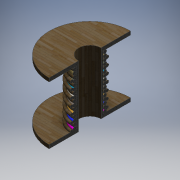
# Autodesk Inventor part: 부품5
Saved by Autodesk Inventor 2016 (Build 200138000, 138)
## iProperties
Created: 2024-06-14
Part Number: 부품5
Material: 강철, 합금
Document SubType Name: Modeling
Designer: pc
Density: 7.73 g/cm^3
Appearance: 내츄럴 단풍나무 - 광택 짙은 착색
Author: pc
Autodesk Inventor part; units mm, degrees
ref_plane "YZ Plane" through (0, 0, 0) normal (1, 0, 0) x (0, 1, 0)
ref_plane "XZ Plane" through (0, 0, 0) normal (0, 1, 0) x (-1, 0, 0)
ref_plane "XY Plane" through (0, 0, 0) normal (0, 0, 1) x (1, 0, 0)
sketch "스케치1" plane through (0, 0, 0) normal (0, 0, 1) x (1, 0, 0)
  circle A0 centre (0, 0) radius 900
  dimension "d0" = 1800
  constraints: 1 centre point, 1 coincident
  measures "d0" diameter of A0
extrude "돌출1" add sketch "스케치1" along normal blind 80
sketch "스케치2" plane through (0, 0, 80) normal (0, 0, 1) x (1, 0, 0)
  circle A0 centre (0, 0) radius 300
  dimension "d3" = 600
  constraints: 1 centre point, 1 coincident
  measures "d3" diameter of A0
extrude "돌출2" add sketch "스케치2" along normal blind 1200
sketch "스케치3" plane through (0, 0, 1280) normal (0, 0, 1) x (1, 0, 0)
  circle A0 centre (0, 0) radius 900
  constraints: 1 centre point, 1 coincident
extrude "돌출3" add sketch "스케치3" along normal blind 80
sketch "스케치4" plane through (0, 0, 1360) normal (0, 0, 1) x (1, 0, 0)
  circle A0 centre (0, 0) radius 250
  dimension "d8" = 500
  constraints: 1 centre point, 1 coincident
  measures "d8" diameter of A0
extrude "돌출4" cut sketch "스케치4" against normal blind 1500
sketch "스케치5" plane through (0, 0, 0) normal (0, 1, 0) x (-1, 0, 0)
  line L0 (0, 2844.7445) -> (0, -1858.6322) construction
  circle A0 centre (-337.5073, 1242.1561) radius 37.8439
  line L1 (-900, 1280) -> (900, 1280) projected
  circle A1 centre (-337.5073, 1166.1561) radius 37.8439
  circle A2 centre (-337.5073, 1090.1561) radius 37.8439
  circle A3 centre (-337.5073, 1014.1561) radius 37.8439
  circle A4 centre (-337.5073, 938.1561) radius 37.8439
  circle A5 centre (-337.5073, 862.1561) radius 37.8439
  circle A6 centre (-337.5073, 786.1561) radius 37.8439
  circle A7 centre (-337.5073, 710.1561) radius 37.8439
  circle A8 centre (-337.5073, 634.1561) radius 37.8439
  circle A9 centre (-337.5073, 558.1561) radius 37.8439
  circle A10 centre (-337.5073, 482.1561) radius 37.8439
  circle A11 centre (-337.5073, 406.1561) radius 37.8439
  circle A12 centre (-337.5073, 330.1561) radius 37.8439
  circle A13 centre (-337.5073, 254.1561) radius 37.8439
  circle A14 centre (-337.5073, 178.1561) radius 37.8439
  circle A15 centre (-337.5073, 102.1561) radius 37.8439
  point P0 (0, 0)
  dimension "d16" = 76
  constraints: 16 centre point, 2 end point, 2 vertical, 1 tangent, 30 other
  measures "d16" distance of A0.centre A1.centre
revolve "회전1" add sketch "스케치5" angle 360 about axis through (0, 0, 2844.7445) along (0, 0, -1)
sketch "스케치6" plane through (0, 0, 0) normal (1, 0, 0) x (0, 1, 0)
  circle A0 centre (-396.9012, 1201.184) radius 32.7676
  point P0 (0, 0)
  constraints: 1 centre point
sketch "스케치7" plane through (0, 0, 0) normal (1, 0, 0) x (0, 1, 0)
  line L0 (0, 1644.2607) -> (-12.7363, -225.4331) construction
  point P0 (0, 0)
  constraints: 2 end point
coil "코일1" sketch "스케치6" operation add axis through (0, 0, 1644.2607) along (0, -0.0068, -1) pitch 160 turns 7 hand left
